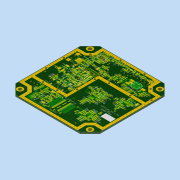
# Autodesk Inventor part: PCB_RX
Saved by Autodesk Inventor 2014 SP1 (Build 180222100, 222)
## iProperties
Created: 2011-02-15
Part Number: PCB_RX
Material: FR4
Document SubType Name: Modeling
Designer: Robert Davis
Mass: 35.4838 g
Surface Area: 181.406 cm^2
Volume: 13.888 cm^3
Density: 2.555 g/cm^3
Appearance: Olive Green
Author: Robert Davis
Autodesk Inventor part; units mm, degrees
sketch "AL_spacer_contact_Zminus" plane through (0, 0, 0) normal (0, 0, 1) x (1, 0, 0)
  circle A0 centre (39.5, 39.5) radius 3.175
  circle A1 centre (39.5, -39.5) radius 3.175
  circle A2 centre (-39.5, -39.5) radius 3.175
  circle A3 centre (-39.5, 39.5) radius 3.175
  point P0 (0, 0)
  dimension "d228" = 39.5
  dimension "d229" = 39.5
  dimension "d230" = 39.5
  dimension "d231" = 39.5
  dimension "d232" = 39.5
  dimension "d233" = 39.5
  dimension "d234" = 39.5
  dimension "d235" = 39.5
  dimension "d236" = 6.35
  constraints: 4 centre point, 3 equal radius
  measures "d228" horizontal distance of point (0, 0) A0.centre
  measures "d229" horizontal distance of point (0, 0) A3.centre
  measures "d230" horizontal distance of point (0, 0) A3.centre
  measures "d231" horizontal distance of point (0, 0) A0.centre
  measures "d232" horizontal distance of A1.centre point (0, 0)
  measures "d233" horizontal distance of point (0, 0) A1.centre
  measures "d234" horizontal distance of point (0, 0) A2.centre
  measures "d235" horizontal distance of point (0, 0) A2.centre
  measures "d236" diameter of A0
sketch "Delrin_stayout_Zminus" plane through (0, 0, 0) normal (0, 0, 1) x (1, 0, 0)
  line L0 (47.5, 39.5) -> (47.5, 31)
  line L1 (47.5, 31) -> (39.5, 31)
  line L2 (39.5, 31) -> (31, 39.5)
  line L3 (31, 39.5) -> (31, 47.5)
  line L4 (31, 47.5) -> (39.5, 47.5)
  line L5 (39.5, 47.5) -> (47.5, 39.5)
  line L6 (-39.5, 47.5) -> (-47.5, 39.5)
  line L7 (-47.5, 39.5) -> (-47.5, 31)
  line L8 (-47.5, 31) -> (-39.5, 31)
  line L9 (-39.5, 31) -> (-31, 39.5)
  line L10 (-31, 39.5) -> (-31, 47.5)
  line L11 (-31, 47.5) -> (-39.5, 47.5)
  line L12 (47.5, -39.5) -> (39.5, -47.5)
  line L13 (39.5, -47.5) -> (31, -47.5)
  line L14 (31, -47.5) -> (31, -39.5)
  line L15 (31, -39.5) -> (39.5, -31)
  line L16 (39.5, -31) -> (47.5, -31)
  line L17 (47.5, -31) -> (47.5, -39.5)
  line L18 (-39.5, -47.5) -> (-47.5, -39.5)
  line L19 (-47.5, -39.5) -> (-47.5, -31)
  line L20 (-47.5, -31) -> (-39.5, -31)
  line L21 (-39.5, -31) -> (-31, -39.5)
  line L22 (-31, -39.5) -> (-31, -47.5)
  line L23 (-31, -47.5) -> (-39.5, -47.5)
  point P0 (0, 0)
  dimension "d243" = 16.5
  dimension "d244" = 8
  dimension "d245" = 8.5
  dimension "d246" = 16.5
  dimension "d247" = 47.5
  dimension "d248" = 47.5
  dimension "d249" = 47.5
  dimension "d250" = 47.5
  dimension "d251" = 47.5
  dimension "d252" = 47.5
  dimension "d253" = 47.5
  dimension "d254" = 47.5
  constraints: 48 end point, 20 equal length, 8 horizontal, 8 vertical
  measures "d243" distance between parallel lines of L3 L0
  measures "d244" distance from line of L4 L0.start
  measures "d245" distance from line of L3 L1.end
  measures "d246" distance between parallel lines of L4 L1
  measures "d247" distance from line of point (0, 0) L0
  measures "d248" distance from line of point (0, 0) L4
  measures "d249" distance from line of L7 point (0, 0)
  measures "d250" distance from line of point (0, 0) L11
  measures "d251" distance from line of point (0, 0) L17
  measures "d252" distance from line of point (0, 0) L13
  measures "d253" distance from line of point (0, 0) L23
  measures "d254" distance from line of point (0, 0) L19
sketch "Nub_stayout_Zminus" plane through (0, 0, 0) normal (0, 0, 1) x (1, 0, 0)
  line L0 (29, 47.5) -> (39.5, 47.5)
  line L1 (39.5, 47.5) -> (47.5, 39.5)
  line L2 (47.5, 39.5) -> (47.5, 29)
  line L3 (47.5, 29) -> (42, 29)
  line L4 (42, 29) -> (42, 40.4125)
  line L5 (40.4125, 42) -> (29, 42)
  line L6 (29, 42) -> (29, 47.5)
  arc A0 (42, 40.4125) -> (40.4125, 42) centre (40.4125, 40.4125) ccw
  line L7 (-29, 47.5) -> (-39.5, 47.5)
  line L8 (-39.5, 47.5) -> (-47.5, 39.5)
  line L9 (-47.5, 39.5) -> (-47.5, 29)
  line L10 (-47.5, 29) -> (-42, 29)
  line L11 (-42, 29) -> (-42, 40.4125)
  line L12 (-40.4125, 42) -> (-29, 42)
  line L13 (-29, 42) -> (-29, 47.5)
  arc A1 (-40.4125, 42) -> (-42, 40.4125) centre (-40.4125, 40.4125) ccw
  line L14 (-47.5, -29) -> (-42, -29)
  line L15 (-42, -29) -> (-42, -40.4125)
  line L16 (-40.4125, -42) -> (-29, -42)
  line L17 (-29, -42) -> (-29, -47.5)
  line L18 (-29, -47.5) -> (-39.5, -47.5)
  line L19 (-39.5, -47.5) -> (-47.5, -39.5)
  line L20 (-47.5, -39.5) -> (-47.5, -29)
  arc A2 (-42, -40.4125) -> (-40.4125, -42) centre (-40.4125, -40.4125) ccw
  line L21 (47.5, -29) -> (42, -29)
  line L22 (42, -29) -> (42, -40.4125)
  line L23 (40.4125, -42) -> (29, -42)
  line L24 (29, -42) -> (29, -47.5)
  line L25 (29, -47.5) -> (39.5, -47.5)
  line L26 (39.5, -47.5) -> (47.5, -39.5)
  line L27 (47.5, -39.5) -> (47.5, -29)
  arc A3 (40.4125, -42) -> (42, -40.4125) centre (40.4125, -40.4125) ccw
  point P0 (0, 0)
  dimension "d255" = 1.5875
  dimension "d256" = 18.5
  dimension "d257" = 8
  dimension "d258" = 5.5
  dimension "d259" = 47.5
  dimension "d260" = 47.5
  dimension "d264" = 1.5875
  dimension "d265" = 47.5
  dimension "d266" = 47.5
  dimension "d267" = 1.5875
  dimension "d268" = 47.5
  dimension "d269" = 47.5
  dimension "d270" = 1.5875
  dimension "d271" = 47.5
  dimension "d272" = 47.5
  constraints: 56 end point, 21 equal length, 12 horizontal, 12 vertical, 8 point on circle, 8 tangent, 4 centre point
  measures "d255" radius of A0
  measures "d256" distance between parallel lines of L6 L2
  measures "d257" distance from line of L2 L0.end
  measures "d258" distance of L5.end L0.start
  measures "d259" distance from line of point (0, 0) L2
  measures "d260" distance from line of point (0, 0) L0
  measures "d264" radius of A1
  measures "d265" distance from line of point (0, 0) L9
  measures "d266" distance from line of point (0, 0) L7
  measures "d267" radius of A2
  measures "d268" distance from line of L18 point (0, 0)
  measures "d269" distance from line of point (0, 0) L20
  measures "d270" radius of A3
  measures "d271" distance from line of point (0, 0) L25
  measures "d272" distance from line of point (0, 0) L27
ref_plane "Zplus_face" through (0, 0, 1.5875) normal (0, 0, 1) x (1, 0, 0)
sketch "AL_spacer_contact_Zplus" plane through (0, 0, 1.5875) normal (0, 0, 1) x (1, 0, 0)
  circle A0 centre (-39.5, 39.5) radius 3.175
  circle A1 centre (-39.5, -39.5) radius 3.175
  circle A2 centre (39.5, -39.5) radius 3.175
  circle A3 centre (39.5, 39.5) radius 3.175
  point P0 (0, 0)
  dimension "d129" = 39.5
  dimension "d130" = 39.5
  dimension "d131" = 39.5
  dimension "d132" = 39.5
  dimension "d133" = 6.35
  constraints: 4 centre point, 3 equal radius, 2 horizontal alignment, 2 vertical alignment
  measures "d129" horizontal distance of A0.centre point (0, 0)
  measures "d130" horizontal distance of point (0, 0) A3.centre
  measures "d131" horizontal distance of point (0, 0) A3.centre
  measures "d132" horizontal distance of point (0, 0) A2.centre
  measures "d133" diameter of A3
sketch "Delrin_stayout_Zplus" plane through (0, 0, 1.5875) normal (0, 0, 1) x (1, 0, 0)
  line L0 (47.5, -31) -> (47.5, -39.5)
  line L1 (47.5, -39.5) -> (39.5, -47.5)
  line L2 (39.5, -47.5) -> (31, -47.5)
  line L3 (31, -47.5) -> (31, -39.5)
  line L4 (31, -39.5) -> (39.5, -31)
  line L5 (39.5, -31) -> (47.5, -31)
  line L6 (47.5, 31) -> (47.5, 39.5)
  line L7 (47.5, 39.5) -> (39.5, 47.5)
  line L8 (39.5, 47.5) -> (31, 47.5)
  line L9 (31, 47.5) -> (31, 39.5)
  line L10 (31, 39.5) -> (39.5, 31)
  line L11 (39.5, 31) -> (47.5, 31)
  line L12 (-39.5, 47.5) -> (-47.5, 39.5)
  line L13 (-47.5, 39.5) -> (-47.5, 31)
  line L14 (-47.5, 31) -> (-39.5, 31)
  line L15 (-39.5, 31) -> (-31, 39.5)
  line L16 (-31, 39.5) -> (-31, 47.5)
  line L17 (-31, 47.5) -> (-39.5, 47.5)
  line L18 (-47.5, -39.5) -> (-39.5, -47.5)
  line L19 (-39.5, -47.5) -> (-31, -47.5)
  line L20 (-31, -47.5) -> (-31, -39.5)
  line L21 (-31, -39.5) -> (-39.5, -31)
  line L22 (-39.5, -31) -> (-47.5, -31)
  line L23 (-47.5, -31) -> (-47.5, -39.5)
  point P0 (0, 0)
  dimension "d115" = 16.5
  dimension "d116" = 16.5
  dimension "d117" = 8
  dimension "d118" = 8.5
  dimension "d121" = 47.5
  dimension "d122" = 47.5
  dimension "d123" = 47.5
  dimension "d124" = 47.5
  dimension "d125" = 47.5
  dimension "d126" = 47.5
  dimension "d127" = 47.5
  dimension "d128" = 47.5
  constraints: 48 end point, 17 equal length, 8 horizontal, 8 vertical, 2 parallel, 1 perpendicular
  measures "d115" distance between parallel lines of L2 L5
  measures "d116" distance between parallel lines of L3 L0
  measures "d117" distance from line of L0 L1.end
  measures "d118" distance from line of L3 L4.end
  measures "d121" distance from line of point (0, 0) L2
  measures "d122" distance from line of point (0, 0) L0
  measures "d123" distance from line of point (0, 0) L8
  measures "d124" distance from line of point (0, 0) L6
  measures "d125" distance from line of point (0, 0) L17
  measures "d126" distance from line of point (0, 0) L13
  measures "d127" distance from line of point (0, 0) L19
  measures "d128" distance from line of point (0, 0) L23
sketch "Nub_stayout_Zplus" plane through (0, 0, 1.5875) normal (0, 0, 1) x (1, 0, 0)
  line L0 (47.5, 29) -> (42, 29)
  line L1 (42, 29) -> (42, 40.4125)
  line L2 (40.4125, 42) -> (29, 42)
  line L3 (29, 42) -> (29, 47.5)
  arc A0 (42, 40.4125) -> (40.4125, 42) centre (40.4125, 40.4125) ccw
  line L4 (29, 47.5) -> (39.5, 47.5)
  line L5 (39.5, 47.5) -> (47.5, 39.5)
  line L6 (47.5, 39.5) -> (47.5, 29)
  line L7 (-39.5, 47.5) -> (-29, 47.5)
  line L8 (-29, 47.5) -> (-29, 42)
  line L9 (-29, 42) -> (-40.4125, 42)
  line L10 (-42, 40.4125) -> (-42, 29)
  line L11 (-42, 29) -> (-47.5, 29)
  line L12 (-47.5, 29) -> (-47.5, 39.5)
  line L13 (-47.5, 39.5) -> (-39.5, 47.5)
  arc A1 (-40.4125, 42) -> (-42, 40.4125) centre (-40.4125, 40.4125) ccw
  line L14 (-47.5, -29) -> (-47.5, -39.5)
  line L15 (-47.5, -39.5) -> (-39.5, -47.5)
  line L16 (-39.5, -47.5) -> (-29, -47.5)
  line L17 (-29, -47.5) -> (-29, -42)
  line L18 (-29, -42) -> (-40.4125, -42)
  line L19 (-42, -40.4125) -> (-42, -29)
  line L20 (-42, -29) -> (-47.5, -29)
  arc A2 (-42, -40.4125) -> (-40.4125, -42) centre (-40.4125, -40.4125) ccw
  line L21 (29, -47.5) -> (39.5, -47.5)
  line L22 (39.5, -47.5) -> (47.5, -39.5)
  line L23 (47.5, -39.5) -> (47.5, -29)
  line L24 (47.5, -29) -> (42, -29)
  line L25 (42, -29) -> (42, -40.4125)
  line L26 (40.4125, -42) -> (29, -42)
  line L27 (29, -42) -> (29, -47.5)
  arc A3 (40.4125, -42) -> (42, -40.4125) centre (40.4125, -40.4125) ccw
  point P0 (0, 0)
  dimension "d146" = 1.5875
  dimension "d147" = 5.5
  dimension "d149" = 18.5
  dimension "d150" = 8
  dimension "d151" = 47.5
  dimension "d152" = 47.5
  dimension "d153" = 1.5875
  dimension "d154" = 47.5
  dimension "d155" = 47.5
  dimension "d156" = 1.5875
  dimension "d157" = 47.5
  dimension "d158" = 47.5
  dimension "d159" = 1.5875
  dimension "d160" = 47.5
  dimension "d161" = 47.5
  constraints: 56 end point, 21 equal length, 12 horizontal, 12 vertical, 8 point on circle, 8 tangent, 4 centre point
  measures "d146" radius of A0
  measures "d147" distance of L0.start L0.end
  measures "d149" distance between parallel lines of L3 L6
  measures "d150" distance from line of L4.end L6
  measures "d151" distance from line of L6 point (0, 0)
  measures "d152" distance from line of point (0, 0) L4
  measures "d153" radius of A1
  measures "d154" distance from line of point (0, 0) L7
  measures "d155" distance from line of point (0, 0) L12
  measures "d156" radius of A2
  measures "d157" distance from line of point (0, 0) L14
  measures "d158" distance from line of point (0, 0) L16
  measures "d159" radius of A3
  measures "d160" distance from line of point (0, 0) L23
  measures "d161" distance from line of point (0, 0) L21
sketch "Sketch1" plane through (0, 0, 0) normal (0, 0, 1) x (1, 0, 0)
  line L0 (-47.5, 47.5) -> (47.5, 47.5)
  line L1 (47.5, 47.5) -> (47.5, -47.5)
  line L2 (47.5, -47.5) -> (-47.5, -47.5)
  line L3 (-47.5, -47.5) -> (-47.5, 47.5)
  point P0 (0, 0)
  dimension "d0" = 95
  dimension "d1" = 95
  dimension "d2" = 47.5
  dimension "d3" = 47.5
  constraints: 8 end point, 2 horizontal, 2 vertical
  measures "d0" distance of L0.start L0.end
  measures "d1" distance of L0.end L1.end
  measures "d2" distance from line of L0 point (0, 0)
  measures "d3" distance from line of L1 point (0, 0)
extrude "Extrusion1" add sketch "Sketch1" along normal blind 1.5875
chamfer "Chamfer2" distance 11 angle 45 4 edges at (-47.5, -47.5, 0.7937) (47.5, -47.5, 0.7937) (47.5, 47.5, 0.7937) (-47.5, 47.5, 0.7937)
ref_plane "Work Plane_ConnX" through (-32, 0, 0) normal (1, 0, 0) x (0, 1, 0)
ref_plane "Work Plane_ConnY" through (0, 0, 0) normal (0, 1, 0) x (-1, 0, 0)
sketch "Sketch9" plane through (0, 0, 1.5875) normal (0, 0, 1) x (1, 0, 0)
  line L0 (47.5, 47.5) -> (47.5, -47.5) projected
  line L1 (58.5598, -32) -> (-58.5598, -32)
  circle A0 centre (-2.667, -21.9289) radius 0.4445
  circle A1 centre (-2.667, -42.0711) radius 0.4445
  line L2 (0, 26.5598) -> (0, -90.5598) construction
  point P0 (0, 0)
  point P1 (0, -32)
  dimension "d134" = 20.1422
  dimension "d136" = 2.667
  dimension "d138" = 0.889
  dimension "d141" = 180
  dimension "d350" = 32
  dimension "d351" = 0
  constraints: 4 end point, 2 centre point, 2 midpoint, 2 perpendicular, 1 symmetric about line, 1 other
  measures "d134" distance of A0.centre A1.centre
  measures "d136" distance from line of L2 A0.centre
  measures "d138" diameter of A0
  measures "d141" angle of L0 L2
  measures "d350" distance of point (0, 0) point (0, -32)
  measures "d351" horizontal distance of point (0, 0) point (0, -32)
extrude "Holes_Conn_Zminus" cut sketch "Sketch9" against normal through all
sketch "Sketch22" plane through (0, 0, 1.5875) normal (0, 0, 1) x (1, 0, 0)
  line L0 (47.5, 36.5) -> (47.5, -36.5) projected
  line L1 (0, -1.0026) -> (0, -62.9974) construction
  line L2 (62.8115, -32) -> (-62.8115, -32)
  circle A0 centre (2.032, -22.7545) radius 0.4445
  circle A1 centre (2.032, -41.2455) radius 0.4445
  point P0 (0, 0)
  point P1 (0, -32)
  dimension "d282" = 180
  dimension "d283" = 18.491
  dimension "d284" = 0.889
  dimension "d285" = 2.032
  dimension "d352" = 32
  dimension "d353" = 0
  constraints: 4 end point, 2 centre point, 2 midpoint, 1 perpendicular, 1 other
  measures "d282" angle of L0 L1
  measures "d283" distance of A0.centre A1.centre
  measures "d284" diameter of A1
  measures "d285" distance from line of L1 A0.centre
  measures "d352" distance of point (0, 0) point (0, -32)
  measures "d353" horizontal distance of point (0, 0) point (0, -32)
extrude "Holes_Conn_Zplus" cut sketch "Sketch22" against normal through all
hole "Hole5" at (39.5, 39.5, 1.5875) direction (0, 0, -1) diameter 3.2 end through all
mirror "Mirror5" about plane through (0, 0, 0) normal (1, 0, 0) of "Hole5"
mirror "Mirror6" about plane through (0, 0, 0) normal (0, 1, 0) of "Hole5", "Mirror5"
sketch "Sketch25" plane through (0, 0, 1.5875) normal (0, 0, 1) x (1, 0, 0)
  circle A0 centre (-39.5, -39.5) radius 1.6 projected
  circle A1 centre (39.5, -39.5) radius 1.6 projected
  circle A2 centre (-39.5, 39.5) radius 1.6 projected
  circle A3 centre (39.5, 39.5) radius 1.6 projected
  line L0 (36.5, -47.5) -> (-36.5, -47.5) projected
  line L1 (0, 0) -> (0, -59.2198)
  line L2 (8, -47.5) -> (8, -15.5)
  line L3 (8, -15.5) -> (-8, -15.5)
  line L4 (-8, -15.5) -> (-8, -47.5)
  line L5 (-8, -47.5) -> (-62.7516, -61.7336)
  line L6 (-62.7516, -61.7336) -> (-64.2933, 68.2222)
  line L7 (-64.2933, 68.2222) -> (58.3572, 62.5728)
  line L8 (58.3572, 62.5728) -> (56.5848, -69.017)
  line L9 (56.5848, -69.017) -> (8, -47.5)
  dimension "d362" = 16
  dimension "d363" = 32
  constraints: 18 end point, 1 coincident, 1 point on line, 1 other
  measures "d362" distance between parallel lines of L2 L4
  measures "d363" distance of L3.end L4.end
extrude "Extrusion9" [suppressed]
sketch "Sketch27" plane through (0, 0, 0) normal (0, 0, -1) x (-1, 0, 0)
  line L0 (36.5, 47.5) -> (-36.5, 47.5) projected
  line L1 (-47.5, 36.5) -> (-47.5, -36.5) projected
  line L2 (-36.5, -47.5) -> (36.5, -47.5) projected
  line L3 (47.5, -36.5) -> (47.5, 36.5) projected
  line L4 (-47.5, 47.5) -> (47.5, 47.5) construction
  line L5 (47.5, 47.5) -> (47.5, -47.5) construction
  line L6 (47.5, -47.5) -> (-47.5, -47.5) construction
  line L7 (-47.5, -47.5) -> (-47.5, 47.5) construction
  point P0 (0, 0)
  constraints: 4 point on line, 2 other
decal "Decal2"
sketch "Sketch29" plane through (0, 0, 1.5875) normal (0, 0, 1) x (1, 0, 0)
  line L0 (-47.5, -36.5) -> (-47.5, 36.5) projected
  line L1 (36.5, -47.5) -> (-36.5, -47.5) projected
  line L2 (47.5, 36.5) -> (47.5, -36.5) projected
  line L3 (-36.5, 47.5) -> (36.5, 47.5) projected
  line L4 (-47.5, 47.5) -> (47.5, 47.5) construction
  line L5 (47.5, 47.5) -> (47.5, -47.5) construction
  line L6 (47.5, -47.5) -> (-47.5, -47.5) construction
  line L7 (-47.5, -47.5) -> (-47.5, 47.5) construction
  point P0 (0, 0)
  constraints: 4 point on line, 2 other
decal "Decal3"
ref_plane "U7_MBC13917_X" through (4.5, -36.5, 0) normal (-1, 0, 0) x (0, 0, 1)
ref_plane "U7_MBC13917_Y" through (-36.5, 42.03, 0) normal (0, -1, 0) x (1, 0, 0)
ref_plane "U9_SA601_X" through (-23.16, -36.5, 0) normal (-1, 0, 0) x (0, 0, 1)
ref_plane "U9_SA601_Y" through (-36.5, 37.32, 0) normal (0, -1, 0) x (1, 0, 0)
ref_plane "U10_SA607_X" through (-18, -36.5, 0) normal (-1, 0, 0) x (0, 0, 1)
ref_plane "U10_SA607_Y" through (-36.5, 4, 0) normal (0, -1, 0) x (1, 0, 0)
hole "Hole13" at (-17.5, -19.5, 1.5875) direction (0, 0, -1) diameter 1.6 end through all
hole "Hole14" at (-7, -7.5, 1.5875) direction (0, 0, -1) diameter 1.6 end through all
hole "Hole15" at (-7, 12.5, 1.5875) direction (0, 0, -1) diameter 1.6 end through all
hole "Hole16" at (5, 16.5, 1.5875) direction (0, 0, -1) diameter 1.6 end through all
hole "Hole17" at (16, 45.5, 1.5875) direction (0, 0, -1) diameter 1.6 end through all
hole "Hole18" at (34, 34.5, 1.5875) direction (0, 0, -1) diameter 1.6 end through all
hole "Hole19" at (45.5, 24, 1.5875) direction (0, 0, -1) diameter 1.6 end through all
hole "Hole20" at (29, 16.5, 1.5875) direction (0, 0, -1) diameter 1.6 end through all
hole "Hole21" at (-11, 45.5, 1.5875) direction (0, 0, -1) diameter 1.6 end through all
hole "Hole22" at (-34, 34.5, 1.5875) direction (0, 0, -1) diameter 1.6 end through all
hole "Hole23" at (-45.5, 16, 1.5875) direction (0, 0, -1) diameter 1.6 end through all
hole "Hole24" at (-45.5, -4, 1.5875) direction (0, 0, -1) diameter 1.6 end through all
hole "Hole25" at (-33.5, -19.5, 1.5875) direction (0, 0, -1) diameter 1.6 end through all
body "Solid1"
